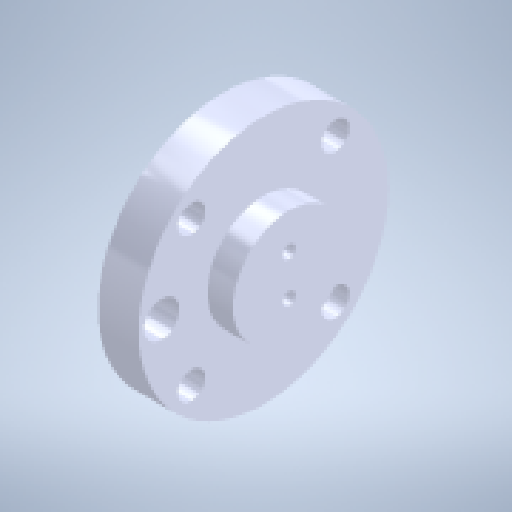
# Autodesk Inventor part: Herramienta Marcador Base
Saved by Autodesk Inventor 2023 (Build 270158000, 158)
## iProperties
Created: 2009-11-11
Part Number: Herramienta Marcador Base
Material: Generic
Document SubType Name: Modeling
Designer: luisd
Density: 1 g/cm^3
Appearance: Default
Sending System: SolidWorks 2011
Last Author: Antonio
Last Saved: 2012-10-30
SAPModified: X
Author: luisd
Autodesk Inventor part; units mm, degrees
ref_plane "YZ Plane" through (0, 0, 0) normal (1, 0, 0) x (0, 1, 0)
ref_plane "XZ Plane" through (0, 0, 0) normal (0, 1, 0) x (-1, 0, 0)
ref_plane "Work Plane1" through (515, 0, 712) normal (1, 0, 0) x (0, 0, -1)
sketch "Sketch1" plane through (515, 0, 712) normal (1, 0, 0) x (0, 0, -1)
  circle A0 centre (0, 0) radius 24.5 projected
  circle A1 centre (0, 0) radius 13.5 projected
  circle A2 centre (14.1421, -14.1421) radius 2.675 projected
  circle A3 centre (14.1421, 14.1421) radius 2.675 projected
  circle A4 centre (-14.1421, 14.1421) radius 2.675 projected
  circle A5 centre (-14.1421, -14.1421) radius 2.675 projected
  arc A6 (-20, 3.5) -> (-20, -3.5) centre (-20, 0) ccw projected
  arc A7 (-20, -3.5) -> (-20, 3.5) centre (-20, 0) ccw projected
  point P0 (712, 0)
extrude "Extrusion1" add sketch "Sketch1" along normal blind 8 contours A0 | A1
sketch "Sketch2" plane through (523, 0, 712) normal (1, 0, 0) x (0, 0, -1)
  circle A0 centre (0, 0) radius 11
  point P0 (712, 0)
  dimension "d2" = 22
  constraints: 1 centre point
  measures "d2" diameter of A0
extrude "Extrusion2" add sketch "Sketch2" along normal blind 5
sketch "Sketch3" plane through (528, 0, 712) normal (1, 0, 0) x (0, 0, -1)
  circle A0 centre (0, -4.0001) radius 1.25
  circle A1 centre (0, 3.9999) radius 1.25
  circle A2 centre (0, 0) radius 11 projected
  point P0 (712, 0)
  dimension "d14" = 8
  dimension "d15" = 22
  constraints: 2 centre point
  measures "d14" distance of A0.centre A1.centre
  measures "d15" diameter of A2
extrude "Extrusion3" cut sketch "Sketch3" against normal blind 3 contours A0 | A1
body "Solid1"
